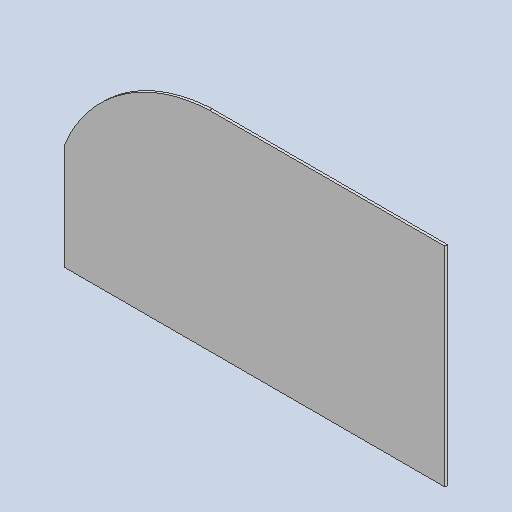
# Autodesk Inventor part: 사이드 카울
Saved by Autodesk Inventor 2025.2 (Build 292293000, 293)
## iProperties
Created: 2025-07-11
Part Number: 사이드 카울
Material: 일반
Document SubType Name: Modeling
Designer: jbhma
Density: 1 g/cm^3
Appearance: 기본값
Author: jbhma
Autodesk Inventor part; units mm, degrees
ref_plane "YZ Plane" through (0, 0, 0) normal (1, 0, 0) x (0, 1, 0)
ref_plane "XZ Plane" through (0, 0, 0) normal (0, 1, 0) x (-1, 0, 0)
ref_plane "XY Plane" through (0, 0, 0) normal (0, 0, 1) x (1, 0, 0)
sketch "스케치1" plane through (0, 0, 0) normal (0, 0, 1) x (1, 0, 0)
  line L0 (552.9734, 795) -> (1450, 795)
  line L1 (1450, 795) -> (1450, 0)
  line L2 (1450, 0) -> (0, 0)
  line L3 (0, 0) -> (0, 405)
  line L4 (0, 0) -> (0, 405) construction
  arc A0 (614, 795) -> (0, 405) centre (583.4867, 164.7107) ccw
  dimension "d0" = 1450
  dimension "d1" = 795
  dimension "d2" = 405
  dimension "d3" = 631.0275
  dimension "d4" = 836
  constraints: 10 end point, 3 point on circle, 2 parallel, 1 centre point, 1 coincident, 1 horizontal, 1 perpendicular, 1 point on line
  measures "d0" distance of L1.end L2.end
  measures "d1" distance of L0.end L1.end
  measures "d2" distance of L3.end L2.end
  measures "d3" radius of A0
  measures "d4" distance from line of A0.start L1
extrude "돌출1" add sketch "스케치1" along normal blind 10 contours L0 L1 L2 L3 A0
